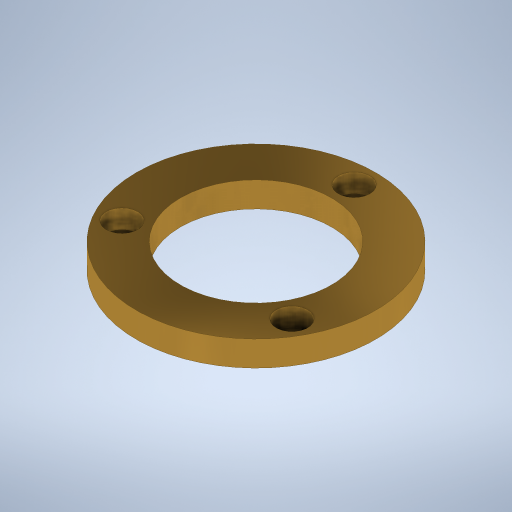
# Autodesk Inventor part: Insert_flange
Saved by Autodesk Inventor 2024 (Build 280153000, 153)
## iProperties
Created: 2023-09-24
Part Number: Insert_flange
Material: Brass
Document SubType Name: Modeling
Designer: schanen
Density: 8.49 g/cm^3
Appearance: Brass - Polished
Author: schanen
Autodesk Inventor part; units mm, degrees
ref_plane "YZ Plane" through (0, 0, 0) normal (1, 0, 0) x (0, 1, 0)
ref_plane "XZ Plane" through (0, 0, 0) normal (0, 1, 0) x (-1, 0, 0)
ref_plane "XY Plane" through (0, 0, 0) normal (0, 0, 1) x (1, 0, 0)
sketch "Sketch1" plane through (0, 0, 0) normal (0, 0, 1) x (1, 0, 0)
  line L0 (-12, 0) -> (-19, 0)
  line L1 (-19, 0) -> (-19, 4)
  line L2 (-19, 4) -> (-12, 4)
  line L3 (-12, 4) -> (-12, 0)
  line L4 (0, -0.8) -> (0, 4.8) projected
  point P0 (0, 0)
  dimension "d0" = 19
  dimension "d1" = 12
  dimension "d2" = 4
  constraints: 8 end point, 2 parallel, 1 horizontal, 1 perpendicular
  measures "d0" distance from line of point (0, 0) L1
  measures "d1" distance from line of point (0, 0) L3
  measures "d2" distance of L0.end L1.end
revolve "Revolution1" add sketch "Sketch1" angle 360 about axis through (0, -10, 0) along (0, 1, 0)
sketch "Sketch3" plane through (0, 4, 0) normal (0, 1, 0) x (1, 0, 0)
  point P0 (0, 0)
  point P1 (0, 15.6)
  dimension "d16" = 15.6
  measures "d16" distance of point (0, 0) point (0, 15.6)
hole "Hole2" at (0, 4, -15.6) direction (0, -1, 0) diameter 3 end through all counterbore diameter 5 counterbore depth 3
pattern_circular "Circular Pattern1" count 3 over 360 about axis through (0, 2, 0) along (0, 1, 0) of "Hole2"
equation "\"d16\" = CD"
equation "\"CD\" = 15.6"
body "Solid1"
